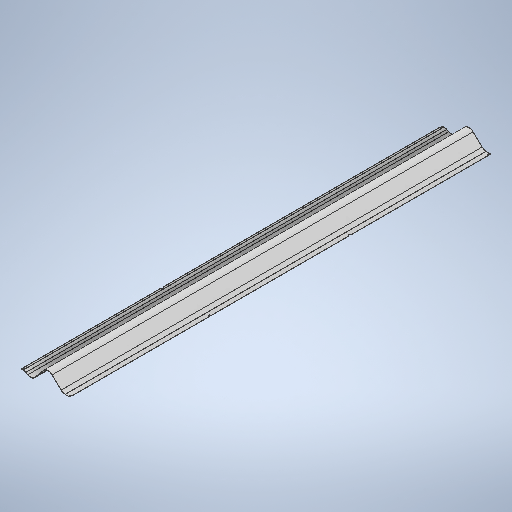
# Autodesk Inventor part: Long_rod
Saved by Autodesk Inventor 2025 (Build 290162000, 162)
## iProperties
Created: 2024-07-10
Part Number: Long_rod
Material: Generic
Document SubType Name: Sheet Metal
Designer: usaid
Density: 1 g/cm^3
Sheet Metal Rule: Default_mm
Appearance: Default
Author: usaid
Autodesk Inventor part; units mm, degrees
ref_plane "YZ Plane" through (0, 0, 0) normal (1, 0, 0) x (0, 1, 0)
ref_plane "XZ Plane" through (0, 0, 0) normal (0, 1, 0) x (-1, 0, 0)
ref_plane "XY Plane" through (0, 0, 0) normal (0, 0, 1) x (1, 0, 0)
sketch "Sketch1" plane through (0, 0, 0) normal (0, 0, 1) x (1, 0, 0)
  line L0 (0, 0) -> (0, -0.7)
  line L1 (0, -0.7) -> (-16.5008, -0.7)
  arc A0 (-30.8857, 5.1157) -> (-16.5008, -0.7) centre (-16.5008, 19.9981) ccw
  line L2 (-30.8857, 5.1157) -> (-62.3007, 35.4806)
  arc A1 (-62.3007, 35.4806) -> (-91.5173, 33.9598) centre (-76.2, 21.1006) ccw
  line L3 (-91.5173, 33.9598) -> (-121.5467, -1.8099)
  arc A2 (-147.1536, -6.7578) -> (-121.5467, -1.8099) centre (-137.3998, 11.4992) ccw
  line L4 (-147.1536, -6.7578) -> (-154.0755, -3.0598)
  arc A3 (-154.0755, -3.0598) -> (-163.5002, -0.7) centre (-163.5002, -20.7009) ccw
  line L5 (-163.5002, -0.7) -> (-170, -0.7)
  line L6 (-170, -0.7) -> (-170, 0)
  line L7 (-170, 0) -> (-163.5, 0)
  arc A4 (-153.747, -2.4419) -> (-163.5, 0) centre (-163.5, -20.6974) ccw
  line L8 (-153.747, -2.4419) -> (-146.8239, -6.1406)
  arc A5 (-146.8239, -6.1406) -> (-122.0828, -1.36) centre (-137.3999, 11.499) ccw
  line L9 (-122.0828, -1.36) -> (-92.0534, 34.4098)
  arc A6 (-61.8138, 35.9838) -> (-92.0534, 34.4098) centre (-76.1998, 21.1004) ccw
  line L10 (-61.8138, 35.9838) -> (-30.3997, 5.6197)
  arc A7 (-30.3997, 5.6197) -> (-16.4996, 0) centre (-16.4996, 20.0004) ccw
  line L11 (-16.4996, 0) -> (0, 0)
  constraints: 24 end point, 16 point on circle, 8 centre point
extrude "Extrusion1" add sketch "Sketch1" along normal mid plane 1470
sketch "Sketch2" plane through (-170, 0, 735) normal (0, 1, 0) x (0, 0, -1)
  line L0 (6.6, -5.2) -> (3.4, -5.2)
  line L1 (3.4, -5.2) -> (3.4, -2)
  line L2 (3.4, -2) -> (6.6, -2)
  line L3 (6.6, -2) -> (6.6, -5.2)
  line L4 (6.6, -5.2) -> (3.4, -2) construction
  line L5 (3.4, -5.2) -> (6.6, -2) construction
  line L6 (1.4, 0) -> (3.4, -2)
  line L7 (3.4, -2) -> (6.6, -2)
  line L8 (6.6, -2) -> (8.6, 0)
  line L9 (8.6, 0) -> (1.4, 0)
  line L10 (493.2667, -5.2) -> (490.0667, -5.2)
  line L11 (490.0667, -5.2) -> (490.0667, -2)
  line L12 (490.0667, -2) -> (493.2667, -2)
  line L13 (493.2667, -2) -> (493.2667, -5.2)
  line L14 (493.2667, -5.2) -> (490.0667, -2) construction
  line L15 (490.0667, -5.2) -> (493.2667, -2) construction
  line L16 (488.0667, 0) -> (490.0667, -2)
  line L17 (490.0667, -2) -> (493.2667, -2)
  line L18 (493.2667, -2) -> (495.2667, 0)
  line L19 (495.2667, 0) -> (488.0667, 0)
  line L20 (979.9333, -5.2) -> (976.7333, -5.2)
  line L21 (976.7333, -5.2) -> (976.7333, -2)
  line L22 (976.7333, -2) -> (979.9333, -2)
  line L23 (979.9333, -2) -> (979.9333, -5.2)
  line L24 (979.9333, -5.2) -> (976.7333, -2) construction
  line L25 (976.7333, -5.2) -> (979.9333, -2) construction
  line L26 (974.7333, 0) -> (976.7333, -2)
  line L27 (976.7333, -2) -> (979.9333, -2)
  line L28 (979.9333, -2) -> (981.9333, 0)
  line L29 (981.9333, 0) -> (974.7333, 0)
  line L30 (1466.6, -5.2) -> (1463.4, -5.2)
  line L31 (1463.4, -5.2) -> (1463.4, -2)
  line L32 (1463.4, -2) -> (1466.6, -2)
  line L33 (1466.6, -2) -> (1466.6, -5.2)
  line L34 (1466.6, -5.2) -> (1463.4, -2) construction
  line L35 (1463.4, -5.2) -> (1466.6, -2) construction
  line L36 (1461.4, 0) -> (1463.4, -2)
  line L37 (1463.4, -2) -> (1466.6, -2)
  line L38 (1466.6, -2) -> (1468.6, 0)
  line L39 (1468.6, 0) -> (1461.4, 0)
  point P0 (5, -3.6)
  point P1 (491.6667, -3.6)
  point P2 (978.3333, -3.6)
  point P3 (1465, -3.6)
  constraints: 80 end point, 8 midpoint, 8 parallel, 4 horizontal, 4 perpendicular
sketch "Sketch3" plane through (0, 0, 735) normal (0, 1, 0) x (0, 0, 1)
  line L0 (-6.6, -5.2) -> (-3.4, -5.2)
  line L1 (-3.4, -5.2) -> (-3.4, -2)
  line L2 (-3.4, -2) -> (-6.6, -2)
  line L3 (-6.6, -2) -> (-6.6, -5.2)
  line L4 (-6.6, -5.2) -> (-3.4, -2) construction
  line L5 (-3.4, -5.2) -> (-6.6, -2) construction
  line L6 (-1.4, 0) -> (-3.4, -2)
  line L7 (-3.4, -2) -> (-6.6, -2)
  line L8 (-6.6, -2) -> (-8.6, 0)
  line L9 (-8.6, 0) -> (-1.4, 0)
  line L10 (-493.2667, -5.2) -> (-490.0667, -5.2)
  line L11 (-490.0667, -5.2) -> (-490.0667, -2)
  line L12 (-490.0667, -2) -> (-493.2667, -2)
  line L13 (-493.2667, -2) -> (-493.2667, -5.2)
  line L14 (-493.2667, -5.2) -> (-490.0667, -2) construction
  line L15 (-490.0667, -5.2) -> (-493.2667, -2) construction
  line L16 (-488.0667, 0) -> (-490.0667, -2)
  line L17 (-490.0667, -2) -> (-493.2667, -2)
  line L18 (-493.2667, -2) -> (-495.2667, 0)
  line L19 (-495.2667, 0) -> (-488.0667, 0)
  line L20 (-979.9333, -5.2) -> (-976.7333, -5.2)
  line L21 (-976.7333, -5.2) -> (-976.7333, -2)
  line L22 (-976.7333, -2) -> (-979.9333, -2)
  line L23 (-979.9333, -2) -> (-979.9333, -5.2)
  line L24 (-979.9333, -5.2) -> (-976.7333, -2) construction
  line L25 (-976.7333, -5.2) -> (-979.9333, -2) construction
  line L26 (-974.7333, 0) -> (-976.7333, -2)
  line L27 (-976.7333, -2) -> (-979.9333, -2)
  line L28 (-979.9333, -2) -> (-981.9333, 0)
  line L29 (-981.9333, 0) -> (-974.7333, 0)
  line L30 (-1466.6, -5.2) -> (-1463.4, -5.2)
  line L31 (-1463.4, -5.2) -> (-1463.4, -2)
  line L32 (-1463.4, -2) -> (-1466.6, -2)
  line L33 (-1466.6, -2) -> (-1466.6, -5.2)
  line L34 (-1466.6, -5.2) -> (-1463.4, -2) construction
  line L35 (-1463.4, -5.2) -> (-1466.6, -2) construction
  line L36 (-1461.4, 0) -> (-1463.4, -2)
  line L37 (-1463.4, -2) -> (-1466.6, -2)
  line L38 (-1466.6, -2) -> (-1468.6, 0)
  line L39 (-1468.6, 0) -> (-1461.4, 0)
  point P0 (-5, -3.6)
  point P1 (-491.6667, -3.6)
  point P2 (-978.3333, -3.6)
  point P3 (-1465, -3.6)
  constraints: 80 end point, 8 midpoint, 8 parallel, 4 horizontal, 4 perpendicular
extrude "Extrusion2" cut sketch "Sketch3" against normal blind 0.7
extrude "Extrusion3" cut sketch "Sketch2" against normal blind 0.7
equation "\"BendRadius\" = Thickness"
equation "\"BendReliefWidth\" = Thickness"
equation "\"BendReliefDepth\" = 0.5 * Thickness"
equation "\"CornerReliefSize\" = 4 * Thickness"
equation "\"MinimumRemnant\" = 2 * Thickness"
equation "\"TransitionRadius\" = BendRadius"
equation "\"JacobiRadiusSize\" = BendRadius"
equation "\"GapSize\" = Thickness"
equation "\"Thickness\" = 0.5"
body "Solid1"
